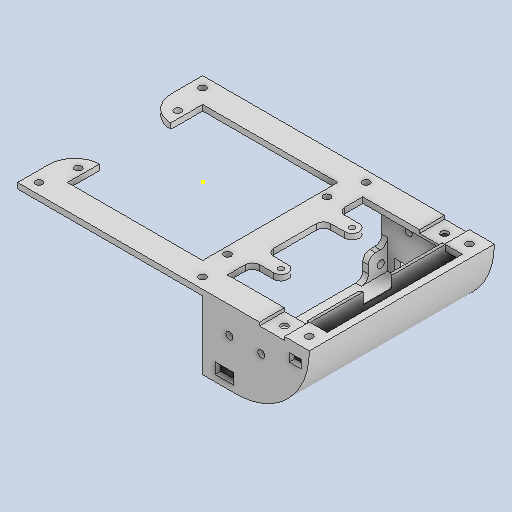
# Autodesk Inventor part: Holder
Saved by Autodesk Inventor 2025 (Build 290162000, 162)
## iProperties
Created: 2025-08-07
Part Number: Holder
Material: Generic
Document SubType Name: Modeling
Designer: Pravoslav
Density: 1 g/cm^3
Appearance: Default
Author: Pravoslav
Autodesk Inventor part; units mm, degrees
ref_plane "YZ Plane" through (0, 0, 0) normal (1, 0, 0) x (0, 1, 0)
ref_plane "XZ Plane" through (0, 0, 0) normal (0, 1, 0) x (-1, 0, 0)
ref_plane "XY Plane" through (0, 0, 0) normal (0, 0, 1) x (1, 0, 0)
sketch "Sketch1" plane through (0, 0, 0) normal (0, 1, 0) x (-1, 0, 0)
  line L0 (57.5, 57.5) -> (-57.5, 57.5)
  line L1 (-57.5, 57.5) -> (-57.5, -57.5)
  line L2 (-57.5, -57.5) -> (57.5, -57.5)
  line L3 (57.5, -57.5) -> (57.5, 57.5)
  line L4 (57.5, 57.5) -> (-57.5, -57.5) construction
  line L5 (-57.5, 57.5) -> (57.5, -57.5) construction
  line L6 (65, 65) -> (-65, 65)
  line L7 (-65, 65) -> (-65, -65)
  line L8 (-65, -65) -> (65, -65)
  line L9 (65, -65) -> (65, 65)
  line L10 (65, 65) -> (-65, -65) construction
  line L11 (-65, 65) -> (65, -65) construction
  line L12 (-65, 65) -> (-50, 65)
  line L13 (-50, 65) -> (-50, 50)
  line L14 (-50, 50) -> (-65, 50)
  line L15 (-65, 50) -> (-65, 65)
  line L16 (65, 65) -> (50, 65)
  line L17 (50, 65) -> (50, 50)
  line L18 (50, 50) -> (65, 50)
  line L19 (65, 50) -> (65, 65)
  line L20 (65, -65) -> (50, -65)
  line L21 (50, -65) -> (50, -50)
  line L22 (50, -50) -> (65, -50)
  line L23 (65, -50) -> (65, -65)
  line L24 (-65, -65) -> (-50, -65)
  line L25 (-50, -65) -> (-50, -50)
  line L26 (-50, -50) -> (-65, -50)
  line L27 (-65, -50) -> (-65, -65)
  circle A0 centre (-57.5, 57.5) radius 2.5
  circle A1 centre (-57.5, -57.5) radius 2.5
  circle A2 centre (57.5, 57.5) radius 2.5
  circle A3 centre (57.5, -57.5) radius 2.5
  point P0 (0, 0)
  point P1 (-50, 57.5)
  point P2 (50, 57.5)
  point P3 (57.5, 50)
  point P4 (57.5, -50)
  point P5 (50, -57.5)
  point P6 (-50, -57.5)
  point P7 (-57.5, -50)
  point P8 (-57.5, 50)
  dimension "d0" = 115
  dimension "d1" = 115
  dimension "d2" = 130
  dimension "d3" = 130
  dimension "d4" = 15
  dimension "d5" = 15
  dimension "d6" = 15
  dimension "d7" = 15
  dimension "d8" = 15
  dimension "d9" = 15
  dimension "d10" = 15
  dimension "d11" = 15
  dimension "d12" = 5
  dimension "d13" = 5
  dimension "d14" = 5
  dimension "d15" = 5
  constraints: 56 end point, 12 parallel, 6 horizontal, 6 perpendicular, 4 centre point, 4 coincident, 4 midpoint
  measures "d0" distance of L2.end L1.end
  measures "d1" distance of L1.end L0.end
  measures "d2" distance of L8.end L7.end
  measures "d3" distance of L7.end L6.end
  measures "d4" distance of L13.end L14.end
  measures "d5" distance of L12.end L13.end
  measures "d6" distance of L18.end L17.end
  measures "d7" distance of L17.end L16.end
  measures "d8" distance of L21.end L22.end
  measures "d9" distance of L20.end L21.end
  measures "d10" distance of L26.end L25.end
  measures "d11" distance of L25.end L24.end
  measures "d12" diameter of A0
  measures "d13" diameter of A1
  measures "d14" diameter of A2
  measures "d15" diameter of A3
extrude "Extrusion1" add sketch "Sketch1" along normal blind 4 contours A0 L1 L14 L7 L6 L13 L0 | L0 L13 L14 L1 A0 | L13 L6 L17 L0 | L17 L6 L9 L18 L3 A2 L0 | L0 A2 L3 L18 L17 | L1 L26 L7 L14 | L26 L25 L2 A1 L1 | L1 A1 L2 L25 L8 L7 L26 | L18 L9 L22 L3 | L22 L9 L8 L21 L2 A3 L3 | L3 A3 L2 L21 L22 | L2 L21 L8 L25
sketch "Sketch2" plane through (0, 4, 0) normal (0, 1, 0) x (1, 0, 0)
  line L0 (-47.5, 47.5) -> (47.5, 47.5)
  line L1 (47.5, 47.5) -> (47.5, -47.5)
  line L2 (47.5, -47.5) -> (-47.5, -47.5)
  line L3 (-47.5, -47.5) -> (-47.5, 47.5)
  line L4 (-47.5, 47.5) -> (47.5, -47.5) construction
  line L5 (47.5, 47.5) -> (-47.5, -47.5) construction
  line L6 (-52.5, 35) -> (52.5, 35)
  line L7 (52.5, 35) -> (52.5, -35)
  line L8 (52.5, -35) -> (-52.5, -35)
  line L9 (-52.5, -35) -> (-52.5, 35)
  line L10 (-52.5, 35) -> (52.5, -35) construction
  line L11 (52.5, 35) -> (-52.5, -35) construction
  circle A0 centre (-52.5, 35) radius 2.5
  circle A1 centre (-52.5, -35) radius 2.5
  circle A2 centre (52.5, -35) radius 2.5
  circle A3 centre (52.5, 35) radius 2.5
  line L12 (-47.5, 47.5) -> (-47.5, 57.8957)
  line L13 (-47.5, 57.8957) -> (-50, 57.8957)
  line L14 (-50, 57.8957) -> (-50, 50)
  line L15 (-57.5, 50) -> (-50, 50) projected
  line L16 (-50, 50) -> (-57.5, 50)
  line L17 (-57.5, 50) -> (-57.5, -50)
  line L18 (-57.5, -50) -> (-50, -50)
  line L19 (-50, -50) -> (-50, -57.5896)
  line L20 (-50, -57.5896) -> (50, -57.5896)
  line L21 (50, -57.5896) -> (50, -50)
  line L22 (50, -50) -> (57.7524, -50)
  line L23 (57.7524, -50) -> (57.7524, 50)
  line L24 (57.7524, 50) -> (50, 50)
  line L25 (50, 50) -> (50, 57.8957)
  line L26 (-47.5, 57.8957) -> (50, 57.8957)
  line L27 (-47.5, 25) -> (-65, 25)
  line L28 (-65, 65) -> (-65, -65) projected
  line L29 (-47.5, -25) -> (-65, -25)
  point P0 (0, 0)
  point P1 (-52.5, 0)
  point P2 (-57.5, -25)
  point P3 (-57.5, 25)
  dimension "d18" = 95
  dimension "d19" = 95
  dimension "d20" = 105
  dimension "d21" = 70
  dimension "d22" = 5
  dimension "d23" = 5
  dimension "d24" = 5
  dimension "d25" = 5
  dimension "d28" = 50
  dimension "d29" = 25
  constraints: 56 end point, 13 point on line, 10 perpendicular, 6 equal length, 5 midpoint, 4 centre point, 4 coincident, 3 horizontal
  measures "d18" distance of L1.end L2.end
  measures "d19" distance of L0.end L1.end
  measures "d20" distance of L7.end L8.end
  measures "d21" distance of L6.end L7.end
  measures "d22" diameter of A0
  measures "d23" diameter of A1
  measures "d24" diameter of A2
  measures "d25" diameter of A3
  measures "d28" distance between parallel lines of L29 L27
  measures "d29" distance from line of L27 point (-52.5, 0)
extrude "Extrusion2" add sketch "Sketch2" against normal blind 4 contours L12 L26 L25 L24 L23 L22 L21 L20 L19 L18 L17 L29 L9 A1 L8 L3 L2 L1 A2 L7 A3 L6 L0 | L3 L6 A0 L9 L27 L17 L15 L14 L13 L12 | L3 L27 L9 A0 L6 | L6 A3 L7 A2 L8 L1 | L3 L29 L9 L27 | L3 L8 A1 L9 L29 | L9 L29 L17 L27 | L17 L29 L28 L27
extrude "Extrusion3" cut sketch "Sketch2" against normal blind 4 contours L3 L29 L9 L27 | L9 L29 L17 L27 | L17 L29 L28 L27
fillet "Fillet1" radius 18 2 edges at (-65, 2, 25) (-65, 2, -25)
sketch "Sketch3" plane through (0, 4, 0) normal (0, 1, 0) x (1, 0, 0)
  line L0 (-65, -65) -> (65, -65) projected
  line L1 (65, -65) -> (140, -65)
  line L2 (140, -65) -> (140, 65)
  line L3 (140, 65) -> (65, 65)
  line L4 (65, 65) -> (65, -65)
  line L5 (65, -65) -> (140, -65)
  line L6 (140, -65) -> (140, -47.5)
  line L7 (140, -47.5) -> (65, -47.5)
  line L8 (65, -47.5) -> (65, -65)
  line L9 (140, -65) -> (122.5, -65)
  line L10 (122.5, -65) -> (122.5, 65)
  line L11 (122.5, 65) -> (140, 65)
  line L12 (140, 65) -> (140, -65)
  line L13 (140, 65) -> (65, 65)
  line L14 (65, 65) -> (65, 47.5)
  line L15 (65, 47.5) -> (140, 47.5)
  line L16 (140, 47.5) -> (140, 65)
  line L17 (122.5, -65) -> (105, -65)
  line L18 (105, -65) -> (105, -47.5)
  line L19 (105, -47.5) -> (122.5, -47.5)
  line L20 (122.5, -47.5) -> (122.5, -65)
  line L21 (122.5, 65) -> (105, 65)
  line L22 (105, 65) -> (105, 47.5)
  line L23 (105, 47.5) -> (122.5, 47.5)
  line L24 (122.5, 47.5) -> (122.5, 65)
  line L25 (65, -30) -> (85, -30)
  line L26 (85, -30) -> (85, 30)
  line L27 (85, 30) -> (65, 30)
  line L28 (65, 30) -> (65, -30)
  circle A0 centre (80, -25) radius 2
  circle A1 centre (80, 25) radius 2
  line L29 (85, -20) -> (65, -20)
  line L30 (65, -20) -> (65, 20)
  line L31 (65, 20) -> (85, 20)
  line L32 (85, 20) -> (85, -20)
  circle A2 centre (131.25, -56.25) radius 2.5
  circle A3 centre (131.25, 56.25) radius 2.5
  circle A4 centre (113.75, -56.25) radius 2.5
  circle A5 centre (113.75, 56.25) radius 2.5
  line L33 (135, -47.5) -> (135, 47.5)
  point P0 (0, 0)
  point P1 (65, 0)
  point P2 (65, 0)
  point P3 (75, 30)
  point P4 (122.5, 56.25)
  dimension "d33" = 75
  dimension "d34" = 130
  dimension "d35" = 17.5
  dimension "d36" = 17.5
  dimension "d37" = 17.5
  dimension "d38" = 17.5
  dimension "d39" = 20
  dimension "d40" = 60
  dimension "d41" = 30
  dimension "d42" = 4
  dimension "d43" = 4
  dimension "d44" = 50
  dimension "d45" = 25
  dimension "d46" = 5
  dimension "d47" = 5
  dimension "d48" = 10
  dimension "d49" = 10
  dimension "d50" = 5
  dimension "d51" = 5
  dimension "d52" = 5
  dimension "d53" = 5
  dimension "d54" = 8.75
  dimension "d55" = 8.75
  dimension "d56" = 8.75
  dimension "d57" = 8.75
  dimension "d58" = 8.75
  dimension "d59" = 8.75
  dimension "d60" = 8.75
  dimension "d61" = 8.75
  dimension "d62" = 17.5
  dimension "d63" = 17.5
  dimension "d64" = 5
  constraints: 66 end point, 16 parallel, 9 perpendicular, 9 point on line, 8 horizontal, 6 centre point, 4 midpoint
  measures "d33" distance of L3.end L2.end
  measures "d34" distance of L2.end L1.end
  measures "d35" distance of L10.end L11.end
  measures "d36" distance of L18.end L19.end
  measures "d37" distance of L23.end L22.end
  measures "d38" distance of L22.end L21.end
  measures "d39" distance of L27.end L26.end
  measures "d40" distance of L26.end L25.end
  measures "d41" distance from line of L25 point (65, 0)
  measures "d42" diameter of A0
  measures "d43" diameter of A1
  measures "d44" distance of A1.centre A0.centre
  measures "d45" vertical distance of point (65, 0) A1.centre
  measures "d46" distance from line of L26 A1.centre
  measures "d47" distance from line of L26 A0.centre
  measures "d48" distance between parallel lines of L25 L29
  measures "d49" distance from line of point (75, 30) L31
  measures "d50" diameter of A2
  measures "d51" diameter of A3
  measures "d52" diameter of A4
  measures "d53" diameter of A5
  measures "d54" distance from line of L1 A2.centre
  measures "d55" distance from line of L10 A2.centre
  measures "d56" distance from line of L1 A4.centre
  measures "d57" distance from line of L18 A4.centre
  measures "d58" distance from line of L15 A3.centre
  measures "d59" distance from line of L24 A3.centre
  measures "d60" distance of point (122.5, 56.25) A5.centre
  measures "d61" distance from line of L15 A5.centre
  measures "d62" distance between parallel lines of L5 L7
  measures "d63" distance between parallel lines of L3 L15
  measures "d64" distance between parallel lines of L2 L33
extrude "Extrusion4" add sketch "Sketch3" against normal blind 4 contours L4 L7 L18 L1 | L18 L7 L10 L1 | L10 L7 L2 L1 | L4 L29 L26 L25 | L7 L33 L15 L2 | L15 L22 L3 L10 | L10 L3 L2 L15 | L4 L27 L26 L31 | L15 L4 L3 L22
fillet "Fillet2" radius 5 8 edges at (65, 2, 30) (65, 2, 20) (85, 2, 30) (85, 2, 20) (65, 2, -20) (85, 2, -20) (85, 2, -30) (65, 2, -30)
sketch "Sketch4" plane through (0, 4, 0) normal (0, 1, 0) x (1, 0, 0)
  point P0 (0, 0)
sketch "Sketch5" plane through (-65, 0, 65) normal (0, 0, 1) x (1, 0, 0)
  circle A0 centre (153, 4) radius 52
  line L0 (205, 4) -> (205, 0) projected
  line L1 (0, 4) -> (205, 4) projected
  line L2 (130, 4) -> (130, 0) projected
  line L3 (130, 4) -> (130, -34.7003)
  line L4 (153, -48) -> (130, -48)
  line L5 (130, 4) -> (130, -48)
  line L6 (0, 0) -> (205, 0) projected
  line L7 (204.8459, 0) -> (205, 0)
  line L8 (205, 0) -> (205, 4)
  point P0 (65, 0)
  point P1 (205, 2)
  point P2 (205, 4)
  point P3 (205, 4)
  dimension "d68" = 104
  dimension "d69" = 52
  dimension "d70" = 0
  constraints: 10 end point, 2 perpendicular, 2 point on circle, 2 point on line, 2 vertical, 1 centre point, 1 collinear, 1 midpoint
  measures "d68" diameter of A0
  measures "d69" horizontal distance of point (205, 2) A0.centre
  measures "d70" distance from line of L1 A0.centre
extrude "Extrusion5" add sketch "Sketch5" against normal blind 4 contours A0 L5 L3 L6 | L4 L5 A0 | L6 L2 L1 A0 picked at (140.8845, -27.2655) picked at (154.9486, 1.3333)
mirror "Mirror1" about plane through (0, 0, 0) normal (0, 0, 1) of "Extrusion5"
sketch "Sketch6" plane through (-65, 0, 61) normal (0, 0, -1) x (-1, 0, 0)
  line L0 (0, 4) -> (-205, 4) projected
  circle A0 centre (-153, 4) radius 50
  line L1 (-205, 4) -> (-205, 0) projected
  line L2 (-153, -46) -> (-130, -46)
  circle A1 centre (-153, 4) radius 52
  line L3 (-130, -48) -> (-153, -48) projected
  line L4 (-153, -48) -> (-130, -48)
  line L5 (-130, -48) -> (-130, -46)
  line L6 (-205, 4) -> (-203, 4)
  point P0 (-65, 0)
  dimension "d75" = 104
  dimension "d73" = 100
  dimension "d74" = 52
  constraints: 8 end point, 2 point on circle, 2 point on line, 1 centre point, 1 coincident, 1 collinear, 1 parallel, 1 perpendicular, 1 tangent, 2 other
  measures "d73" diameter of A0
  measures "d74" distance from line of A0.centre L1
extrude "Extrusion6" add sketch "Sketch6" along normal up to surface (122 mm away) contours L0 A0 L2 A1 | L2 L5 L3 A1 picked at (-191.921, -28.1863)
extrude "Extrusion7" cut sketch "Sketch5" against normal through all contours A0 L0 L6
sketch "Sketch7" plane through (65, -48, -65) normal (-1, 0, 0) x (0, 0, 1)
  line L0 (0, 48) -> (0, 0) projected
  line L1 (0, 0) -> (17.5, 0)
  line L2 (17.5, 0) -> (17.5, 17.5)
  line L3 (17.5, 17.5) -> (0, 17.5)
  line L4 (0, 17.5) -> (0, 0)
  line L5 (130, 48) -> (130, 0) projected
  line L6 (130, 0) -> (112.5, 0)
  line L7 (112.5, 0) -> (112.5, 17.5)
  line L8 (112.5, 17.5) -> (130, 17.5)
  line L9 (130, 17.5) -> (130, 0)
  circle A0 centre (121.25, 8.75) radius 2.5
  circle A1 centre (8.75, 8.75) radius 2.5
  point P0 (65, 48)
  point P1 (8.75, 17.5)
  point P2 (130, 17.5)
  dimension "d80" = 17.5
  dimension "d81" = 17.5
  dimension "d82" = 17.5
  dimension "d83" = 17.5
  dimension "d84" = 5
  dimension "d85" = 5
  dimension "d86" = 8.75
  dimension "d87" = 8.75
  dimension "d88" = 8.75
  dimension "d89" = 8.75
  constraints: 16 end point, 4 parallel, 2 centre point, 2 horizontal, 2 perpendicular, 1 midpoint
  measures "d80" distance of L3.end L2.end
  measures "d81" distance of L2.end L1.end
  measures "d82" distance of L7.end L8.end
  measures "d83" distance between parallel lines of L6 L8
  measures "d84" diameter of A0
  measures "d85" diameter of A1
  measures "d86" distance of point (8.75, 17.5) A1.centre
  measures "d87" distance from line of L0 A1.centre
  measures "d88" distance from line of L8 A0.centre
  measures "d89" distance from line of L7 A0.centre
extrude "Extrusion8" add sketch "Sketch7" against normal blind 4
fillet "Fillet3" radius 5 6 edges at (67, -30.5, 47.5) (67, -30.5, -47.5) (67, -30.5, 61) (67, -46, 47.5) (67, -46, -47.5) (67, -30.5, -61)
sketch "Sketch8" plane through (0, 4, 0) normal (0, 1, 0) x (1, 0, 0)
  line L0 (65, 47.5) -> (135, 47.5) projected
  line L1 (135, -47.5) -> (65, -47.5) projected
  line L2 (121, 47.5) -> (123, 47.5)
  line L3 (123, 47.5) -> (123, -47.5)
  line L4 (123, -47.5) -> (121, -47.5)
  line L5 (121, -47.5) -> (121, 47.5)
  line L6 (140, -65) -> (140, 65) projected
  line L7 (140, 65) -> (-65, 65) projected
  line L8 (121, 47.5) -> (123, 47.5)
  line L9 (123, 47.5) -> (123, 65)
  line L10 (123, 65) -> (121, 65)
  line L11 (121, 65) -> (121, 47.5)
  line L12 (121, -47.5) -> (123, -47.5)
  line L13 (123, -47.5) -> (123, -65)
  line L14 (123, -65) -> (121, -65)
  line L15 (121, -65) -> (121, -47.5)
  point P0 (0, 0)
  point P1 (123, -47.5)
  dimension "d93" = 2
  dimension "d94" = 17
  constraints: 24 end point, 6 parallel, 4 point on line, 3 horizontal, 3 perpendicular
  measures "d93" distance of L3.end L4.end
  measures "d94" distance between parallel lines of L6 L3
extrude "Extrusion9" add sketch "Sketch8" against normal up to surface round surface about axis through (88, 4, 61) along (0, 0, -1) radius 50 far side no
sketch "Sketch9" plane through (121, 4, -47.5) normal (-1, 0, 0) x (0, 0, 1)
  line L0 (112.5, 0) -> (-17.5, 0) projected
  line L1 (37.5, 0) -> (57.5, 0)
  line L2 (57.5, -4) -> (37.5, -4)
  line L3 (37.5, 0) -> (57.5, 0)
  line L4 (57.5, 0) -> (57.5, -10)
  line L5 (57.5, -10) -> (37.5, -10)
  line L6 (37.5, -10) -> (37.5, 0)
  line L7 (37.5, -4) -> (57.5, -4)
  line L8 (57.5, -4) -> (57.5, -8)
  line L9 (57.5, -8) -> (37.5, -8)
  line L10 (37.5, -8) -> (37.5, -4)
  point P0 (47.5, -4)
  point P1 (47.5, -4)
  dimension "d97" = 20
  dimension "d126" = 10
  dimension "d127" = 4
  constraints: 20 end point, 5 parallel, 3 horizontal, 2 perpendicular, 2 point on line
  measures "d97" distance of L2.start L2.end
  measures "d126" distance of L3.end L4.end
  measures "d127" distance of L7.end L8.end
extrude "Extrusion10" cut sketch "Sketch9" against normal up to surface (2 mm away) contours L4 L2 L6 L0 | L4 L9 L6 L2
fillet "Fillet4" radius 2 3 edges at (121, 0, -10) (121, -4, 0) (121, 0, 10)
sketch "Sketch10" plane through (0, 4, 0) normal (0, 1, 0) x (1, 0, 0)
  line L0 (140, 65) -> (-65, 65) projected
  line L1 (105, 65) -> (122.5, 65)
  line L2 (122.5, 65) -> (122.5, 47.5)
  line L3 (122.5, 47.5) -> (105, 47.5)
  line L4 (105, 47.5) -> (105, 65)
  line L5 (121, -47.5) -> (65, -47.5) projected
  line L6 (105, -47.5) -> (122.5, -47.5)
  line L7 (122.5, -47.5) -> (122.5, -65)
  line L8 (122.5, -65) -> (105, -65)
  line L9 (105, -65) -> (105, -47.5)
  circle A0 centre (113.75, 56.25) radius 2.5 projected
  circle A1 centre (113.75, -56.25) radius 2.5 projected
  point P0 (0, 0)
  point P1 (122.5, -56.25)
  dimension "d102" = 17.5
  dimension "d103" = 17.5
  dimension "d104" = 17.5
  dimension "d105" = 17.5
  dimension "d106" = 8.75
  dimension "d107" = 8.75
  constraints: 16 end point, 4 parallel, 2 horizontal, 2 perpendicular, 2 point on line, 1 midpoint
  measures "d102" distance of L2.end L3.end
  measures "d103" distance of L7.end L8.end
  measures "d104" distance of L6.end L7.end
  measures "d105" distance between parallel lines of L0 L3
  measures "d106" distance from line of L2 A0.centre
  measures "d107" distance of A1.centre point (122.5, -56.25)
extrude "Extrusion11" cut sketch "Sketch10" against normal blind 2.3
sketch "Sketch11" plane through (-65, 0, 61) normal (0, 0, -1) x (-1, 0, 0)
  line L0 (-186, 0) -> (-186, -33.5633) projected
  line L1 (-188, -31.7071) -> (-188, 0) projected
  arc A0 (-202.8397, 0) -> (-188, -31.7071) centre (-153, 4) ccw projected
  arc A1 (-205, 4) -> (-153, -48) centre (-153, 4) ccw projected
  line L2 (-153, -46) -> (-134, -46) projected
  line L3 (-134, -46) -> (-134, -25.5) projected
  line L4 (-130, -25.5) -> (-130, 0) projected
  line L5 (-130, -25.5) -> (-134, -25.5) projected
  line L6 (-130, 0) -> (-186, 0) projected
  arc A2 (-186, -33.5633) -> (-153, -46) centre (-153, 4) ccw projected
  line L7 (-199.3636, -3.9865) -> (-190.7736, -3.9865)
  line L8 (-190.7736, -3.9865) -> (-190.7736, -9.8792)
  line L9 (-190.7736, -9.8792) -> (-199.3636, -9.8792)
  line L10 (-199.3636, -9.8792) -> (-199.3636, -3.9865)
  line L11 (-151.8317, -35.75) -> (-138.7846, -35.75)
  line L12 (-138.7846, -35.75) -> (-138.7846, -43.4217)
  line L13 (-138.7846, -43.4217) -> (-151.8317, -43.4217)
  line L14 (-151.8317, -43.4217) -> (-151.8317, -35.75)
  line L15 (-180, -6) -> (-162.5, -6)
  line L16 (-162.5, -6) -> (-162.5, -23.5)
  line L17 (-162.5, -23.5) -> (-180, -23.5)
  line L18 (-180, -23.5) -> (-180, -6)
  line L19 (-157.5, -6) -> (-140, -6)
  line L20 (-140, -6) -> (-140, -23.5)
  line L21 (-140, -23.5) -> (-157.5, -23.5)
  line L22 (-157.5, -23.5) -> (-157.5, -6)
  line L23 (0, 4) -> (-170, 4) projected
  circle A3 centre (-171.25, -14.75) radius 2.5
  circle A4 centre (-148.75, -14.75) radius 2.5
  point P0 (-65, 0)
  point P1 (-157.8422, -11.1136)
  point P2 (-139.6865, -13.9382)
  point P3 (-148.75, -23.5)
  dimension "d110" = 17.5
  dimension "d111" = 17.5
  dimension "d112" = 17.5
  dimension "d113" = 17.5
  dimension "d114" = 5
  dimension "d115" = 10
  dimension "d116" = 10
  dimension "d117" = 10
  dimension "d118" = 5
  dimension "d119" = 5
  dimension "d120" = 8.75
  dimension "d121" = 8.75
  dimension "d122" = 8.75
  dimension "d123" = 8.75
  constraints: 32 end point, 8 parallel, 4 horizontal, 4 perpendicular, 2 centre point, 1 midpoint
  measures "d110" distance of L16.end L17.end
  measures "d111" distance of L15.end L16.end
  measures "d112" distance of L21.start L21.end
  measures "d113" distance of L19.end L21.start
  measures "d114" distance between parallel lines of L22 L16
  measures "d115" distance between parallel lines of L23 L15
  measures "d116" distance between parallel lines of L23 L19
  measures "d117" distance between parallel lines of L4 L20
  measures "d118" diameter of A3
  measures "d119" diameter of A4
  measures "d120" distance from line of L19 A4.centre
  measures "d121" distance of point (-148.75, -23.5) A4.centre
  measures "d122" distance from line of L15 A3.centre
  measures "d123" distance from line of L18 A3.centre
extrude "Extrusion12" cut sketch "Sketch11" against normal through all contours L7 L8 L9 L10 | L11 L12 L13 L14 | A3 | A4
mirror "Mirror2" about plane through (0, 0, 0) normal (0, 0, 1) of "Extrusion12"
body "Solid1"
